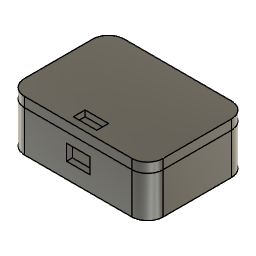
caseAlimentazione (Autodesk Fusion 360 design; units mm, degrees)
Autodesk Fusion 360 part; units mm, degrees
note: some values were not read from the file. Set by a fixed rule: which face or edge a step refers to.
sketch "Schizzo1" plane through (0, 0, 0) normal (0, 0, 1) x (1, 0, 0)
  line L0 (32.5, 22.5) -> (-32.5, 22.5)
  line L1 (-32.5, 22.5) -> (-32.5, -22.5)
  line L2 (-32.5, -22.5) -> (32.5, -22.5)
  line L3 (32.5, -22.5) -> (32.5, 22.5)
  line L4 (32.5, 22.5) -> (-32.5, -22.5) construction
  line L5 (-32.5, 22.5) -> (32.5, -22.5) construction
  dimension "d1" = 65
  dimension "d2" = 45
  constraint horizontal L0
  constraint perpendicular L0 L1
  constraint parallel L0 L2
  constraint parallel L1 L3
  constraint coincident L4 origin
  constraint coincident L5 origin
  measures "d1" distance of L1.end L2.end
  measures "d2" distance of L0.end L1.end
extrude "Estrusione1" add sketch "Schizzo1" along normal blind 20 makes body 1
fillet "Raccordo1" radius 5 4 edges at (-32.5, -22.5, 10) (-32.5, 22.5, 10) (32.5, 22.5, 10) (32.5, -22.5, 10) on bodies 1
shell "Shell1" thickness 3 outward yes removed faces 0 bodies 1
sketch "Schizzo3" plane through (-35.5, 0, 0) normal (-1, 0, 0) x (0, -1, 0)
  line L0 (-17.5, 23) -> (-17.5, -3)
  line L1 (-17.5, -3) -> (17.5, -3)
  line L2 (17.5, -3) -> (17.5, 23)
  line L3 (2.5, 19.5) -> (-2.5, 19.5)
  line L4 (-2.5, 19.5) -> (-2.5, 16)
  line L5 (-2.5, 16) -> (2.5, 16)
  line L6 (2.5, 16) -> (2.5, 19.5)
  line L7 (2.5, 19.5) -> (-2.5, 16) construction
  line L8 (-2.5, 19.5) -> (2.5, 16) construction
  line L9 (17.5, 23) -> (-17.5, 23)
  point P0 (0, 17.75)
  dimension "d33" = 5
  dimension "d34" = 3.5
  constraint horizontal L3
  constraint perpendicular L3 L4
  constraint parallel L3 L5
  constraint parallel L4 L6
  constraint coincident L7 P0
  constraint coincident L8 P0
  measures "d33" distance of L4.end L5.end
  measures "d34" distance of L3.end L4.end
extrude "Estrusione3" cut sketch "Schizzo3" against normal up to surface (3 mm away) contours L3 L4 L5 L6 bodies 1
sketch "Schizzo4" plane through (0, -25.5, 0) normal (0, -1, 0) x (1, 0, 0)
  line L0 (-27.5, 23) -> (-27.5, -3)
  line L1 (-27.5, -3) -> (27.5, -3)
  line L2 (27.5, -3) -> (27.5, 23)
  line L3 (27.5, 23) -> (-27.5, 23)
  line L4 (-6, 5) -> (6, 5)
  line L5 (6, 5) -> (6, 13)
  line L6 (6, 13) -> (-6, 13)
  line L7 (-6, 13) -> (-6, 5)
  dimension "d37" = 12
  dimension "d38" = 8
  constraint horizontal L4
  constraint vertical L5
  constraint horizontal L6
  constraint vertical L7
  measures "d37" distance of L4.start L4.end
  measures "d38" distance of L4.start L6.end
extrude "Estrusione4" cut sketch "Schizzo4" against normal blind 3 contours L4 L5 L6 L7 bodies 1
move_body "Sposta1" bodies 1 to x (1, 0, 0) y (0, 1, 0) z (0, 0, 1) at (0, 0, 3)
sketch "Schizzo5" plane through (0, 0, 26) normal (0, 0, 1) x (-1, 0, 0)
  arc A0 (-27.5, 25.5) -> (-35.5, 17.5) centre (-27.5, 17.5) ccw
  line L0 (-35.5, 17.5) -> (-35.5, -17.5)
  arc A1 (-35.5, -17.5) -> (-27.5, -25.5) centre (-27.5, -17.5) ccw
  line L1 (-27.5, -25.5) -> (27.5, -25.5)
  arc A2 (27.5, -25.5) -> (35.5, -17.5) centre (27.5, -17.5) ccw
  line L2 (35.5, -17.5) -> (35.5, 17.5)
  arc A3 (35.5, 17.5) -> (27.5, 25.5) centre (27.5, 17.5) ccw
  line L3 (27.5, 25.5) -> (-27.5, 25.5)
  line L4 (6, 22) -> (-6, 22)
  line L5 (-6, 22) -> (-6, 16)
  line L6 (-6, 16) -> (6, 16)
  line L7 (6, 16) -> (6, 22)
  constraint horizontal L4
  constraint vertical L5
  constraint horizontal L6
  constraint vertical L7
extrude "Estrusione5" cut sketch "Schizzo5" against normal blind 3 contours L4 L5 L6 L7 bodies 1
sketch "Schizzo9" plane through (0, 25.5, 0) normal (0, 1, 0) x (-1, 0, 0)
  line L0 (-27.5, 26) -> (-27.5, 0)
  line L1 (-27.5, 0) -> (27.5, 0)
  line L2 (27.5, 0) -> (27.5, 26)
  line L3 (27.5, 26) -> (-27.5, 26)
  circle A0 centre (0, 15) radius 5
  dimension "d51" = 10
  dimension "d71" = 15
  measures "d51" diameter of A0
  measures "d71" distance of L1 A0.centre
extrude "Estrusione7" cut sketch "Schizzo9" against normal up to surface (3 mm away) contours A0 bodies 1
ref_plane "Piano di lavoro3" through (0, 0, 21) normal (0, 0, 1) x (1, 0, 0)
split "Dividi2" by plane through (0, 0, 21) normal (0, 0, 1) bodies 1 makes body 2 at (2, 11.6667, 26)
sketch "Schizzo10" plane through (0, 0, 3) normal (0, 0, 1) x (-1, 0, 0)
  arc A0 (-27.5, 22.5) -> (-32.5, 17.5) centre (-27.5, 17.5) ccw
  line L0 (-32.5, 17.5) -> (-32.5, -17.5)
  arc A1 (-32.5, -17.5) -> (-27.5, -22.5) centre (-27.5, -17.5) ccw
  line L1 (-27.5, -22.5) -> (27.5, -22.5)
  arc A2 (27.5, -22.5) -> (32.5, -17.5) centre (27.5, -17.5) ccw
  line L2 (32.5, -17.5) -> (32.5, 17.5)
  arc A3 (32.5, 17.5) -> (27.5, 22.5) centre (27.5, 17.5) ccw
  line L3 (27.5, 22.5) -> (-27.5, 22.5)
  circle A4 centre (27, -18) radius 1.5
  circle A5 centre (27, 18.5) radius 1.5
  circle A6 centre (-29.1, 18) radius 1.5
  circle A7 centre (-29.2, -18) radius 1.5
  circle A8 centre (27, -18) radius 3
  circle A9 centre (27, 18.5) radius 3
  circle A10 centre (-29.1, 18) radius 2.5
  circle A11 centre (-29.2, -18) radius 2.5
  dimension "d54" = 3
  dimension "d55" = 3
  dimension "d56" = 3
  dimension "d57" = 3
  dimension "d58" = 6
  dimension "d59" = 6
  dimension "d60" = 5
  dimension "d61" = 5
  constraint concentric A4 A8
  constraint concentric A5 A9
  constraint concentric A6 A10
  constraint concentric A7 A11
  measures "d54" diameter of A4
  measures "d55" diameter of A5
  measures "d56" diameter of A6
  measures "d57" diameter of A7
  measures "d58" diameter of A8
  measures "d59" diameter of A9
  measures "d60" diameter of A10
  measures "d61" diameter of A11
extrude "Estrusione8" add sketch "Schizzo10" along normal blind 3.5 contours A8 | A9 | A10 | A11 bodies 1
sketch "Schizzo17" plane through (0, 0, 21) normal (0, 0, 1) x (-1, 0, 0)
  line L0 (34.5, 3.5) -> (34.5, 17.5)
  arc A0 (34.5, 17.5) -> (27.5, 24.5) centre (27.5, 17.5) ccw
  line L1 (27.5, 24.5) -> (-27.5, 24.5)
  arc A1 (-27.5, 24.5) -> (-34.5, 17.5) centre (-27.5, 17.5) ccw
  line L2 (-34.5, 17.5) -> (-34.5, -17.5)
  arc A2 (-34.5, -17.5) -> (-27.5, -24.5) centre (-27.5, -17.5) ccw
  line L3 (-27.5, -24.5) -> (27.5, -24.5)
  arc A3 (27.5, -24.5) -> (34.5, -17.5) centre (27.5, -17.5) ccw
  line L4 (34.5, -17.5) -> (34.5, -3.5)
  line L5 (34.5, -3.5) -> (33.5, -3.5)
  line L6 (33.5, -3.5) -> (33.5, -17.5)
  arc A4 (27.5, -23.5) -> (33.5, -17.5) centre (27.5, -17.5) ccw
  line L7 (27.5, -23.5) -> (-27.5, -23.5)
  arc A5 (-33.5, -17.5) -> (-27.5, -23.5) centre (-27.5, -17.5) ccw
  line L8 (-33.5, -17.5) -> (-33.5, 17.5)
  arc A6 (-27.5, 23.5) -> (-33.5, 17.5) centre (-27.5, 17.5) ccw
  line L9 (-27.5, 23.5) -> (27.5, 23.5)
  arc A7 (33.5, 17.5) -> (27.5, 23.5) centre (27.5, 17.5) ccw
  line L10 (33.5, 17.5) -> (33.5, 3.5)
  line L11 (33.5, 3.5) -> (34.5, 3.5)
  arc A8 (-27.5, 22.5) -> (-32.5, 17.5) centre (-27.5, 17.5) ccw
  line L12 (-27.5, 22.5) -> (27.5, 22.5)
  arc A9 (32.5, 17.5) -> (27.5, 22.5) centre (27.5, 17.5) ccw
  line L13 (32.5, -2.5) -> (32.5, -17.5)
  arc A10 (27.5, -22.5) -> (32.5, -17.5) centre (27.5, -17.5) ccw
  line L14 (27.5, -22.5) -> (-27.5, -22.5)
  arc A11 (-32.5, -17.5) -> (-27.5, -22.5) centre (-27.5, -17.5) ccw
  line L15 (-32.5, -17.5) -> (-32.5, 17.5)
  arc A12 (-27.5, 25.5) -> (-35.5, 17.5) centre (-27.5, 17.5) ccw
  line L16 (-35.5, 17.5) -> (-35.5, -17.5)
  arc A13 (-35.5, -17.5) -> (-27.5, -25.5) centre (-27.5, -17.5) ccw
  line L17 (-27.5, -25.5) -> (27.5, -25.5)
  arc A14 (27.5, -25.5) -> (35.5, -17.5) centre (27.5, -17.5) ccw
  line L18 (35.5, -17.5) -> (35.5, -2.5)
  arc A15 (35.5, 17.5) -> (27.5, 25.5) centre (27.5, 17.5) ccw
  line L19 (27.5, 25.5) -> (-27.5, 25.5)
  line L20 (35.5, -2.5) -> (32.5, -2.5)
  line L21 (32.5, 17.5) -> (32.5, 2.5)
  line L22 (32.5, 2.5) -> (35.5, 2.5)
  line L23 (35.5, 2.5) -> (35.5, 17.5)
  constraint tangent A0 L1
  constraint tangent L0 A0
  constraint tangent L1 A1
  constraint tangent A1 L2
  constraint tangent L3 A3
  constraint tangent L2 A2
  constraint tangent A2 L3
  constraint tangent A3 L4
  constraint tangent L6 A4
  constraint tangent A4 L7
  constraint tangent L7 A5
  constraint tangent A5 L8
  constraint tangent L8 A6
  constraint tangent A6 L9
  constraint tangent L9 A7
  constraint tangent A7 L10
extrude "Estrusione10" add sketch "Schizzo17" along normal blind 2.5 contours L0 A0 L1 A1 L2 A2 L3 A3 L4 L5 L6 A4 L7 A5 L8 A6 L9 A7 L10 L11 bodies 1
fillet "Raccordo4" radius 0.5 18 edges at (-33.5, 10.5, 23.5) (-31.7426, 21.7426, 23.5) (0, 23.5, 23.5) (31.7426, 21.7426, 23.5) (33.5, 0, 23.5) (31.7426, -21.7426, 23.5) (0, -23.5, 23.5) (-31.7426, -21.7426, 23.5) (-33.5, -10.5, 23.5) (-34.5, -10.5, 23.5) (-32.4497, -22.4497, 23.5) (0, -24.5, 23.5) (32.4497, -22.4497, 23.5) (34.5, 0, 23.5) (32.4497, 22.4497, 23.5) (0, 24.5, 23.5) (-32.4497, 22.4497, 23.5) (-34.5, 10.5, 23.5) on bodies 1
combine "Combina3" operation cut target body 2 tool bodies 1 keep tools
